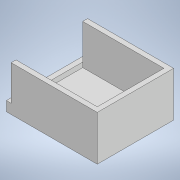
# Autodesk Inventor part: Z Fold Jig
Saved by Autodesk Inventor 2022 (Build 260153000, 153)
## iProperties
Created: 2022-03-05
Part Number: Z Fold Jig
Material: Generic
Document SubType Name: Modeling
Designer: Nick
Density: 1 g/cm^3
Appearance: Default
Author: Nick
Autodesk Inventor part; units mm, degrees
ref_plane "YZ Plane" through (0, 0, 0) normal (1, 0, 0) x (0, 1, 0)
ref_plane "XZ Plane" through (0, 0, 0) normal (0, 1, 0) x (-1, 0, 0)
ref_plane "XY Plane" through (0, 0, 0) normal (0, 0, 1) x (1, 0, 0)
sketch "Sketch1" plane through (0, 0, 0) normal (0, 1, 0) x (-1, 0, 0)
  line L0 (0, 0) -> (67, 0)
  line L1 (67, 0) -> (67, -55)
  line L2 (67, -55) -> (0, -55)
  line L3 (0, -55) -> (0, 0)
  line L4 (-4, -59) -> (71, -59)
  line L5 (71, -59) -> (71, 4)
  line L6 (71, 4) -> (-4, 4)
  line L7 (-4, 4) -> (-4, -59)
  line L8 (67, 4) -> (67, -59)
  dimension "d0" = 67
  dimension "d1" = 55
  dimension "d2" = 4
  constraints: 18 end point, 4 parallel, 2 perpendicular, 2 point on line, 1 collinear, 1 horizontal, 1 vertical, 3 other
  measures "d0" distance of L1.end L2.end
  measures "d1" distance of L0.end L1.end
  measures "d2" distance between parallel lines of L2 L4
extrude "Extrusion1" add sketch "Sketch1" along normal blind 33 contours L3 L2 L8 L4 L7 L6 L0
extrude "Extrusion2" add sketch "Sketch1" against normal blind 4
extrude "Extrusion3" add sketch "Sketch1" along normal blind 4 contours L8 L6 L5 L4 L1
body "Solid1"
